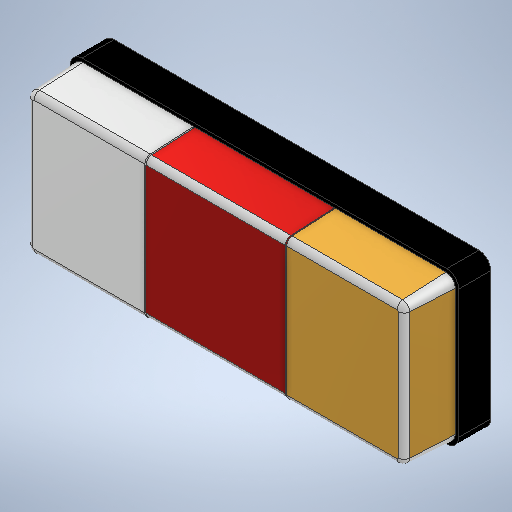
# Autodesk Inventor part: Arjun_RearLight
Saved by Autodesk Inventor 2025 (Build 290162000, 162)
## iProperties
Created: 2024-11-03
Part Number: Arjun_RearLight
Material: Generic
Document SubType Name: Modeling
Designer: pathl
Density: 1 g/cm^3
Appearance: Default
Author: pathl
Autodesk Inventor part; units mm, degrees
ref_plane "YZ Plane" through (0, 0, 0) normal (1, 0, 0) x (0, 1, 0)
ref_plane "XZ Plane" through (0, 0, 0) normal (0, 1, 0) x (-1, 0, 0)
ref_plane "XY Plane" through (0, 0, 0) normal (0, 0, 1) x (1, 0, 0)
sketch "Sketch1" plane through (0, 0, 0) normal (0, 0, 1) x (1, 0, 0)
  line L0 (7, 90) -> (223, 90)
  line L1 (230, 83) -> (230, 7)
  line L2 (223, 0) -> (7, 0)
  line L3 (0, 7) -> (0, 83)
  arc A0 (0, 7) -> (7, 0) centre (7, 7) ccw
  arc A1 (7, 90) -> (0, 83) centre (7, 83) ccw
  arc A2 (230, 83) -> (223, 90) centre (223, 83) ccw
  arc A3 (223, 0) -> (230, 7) centre (223, 7) ccw
  point P0 (0, 0)
  point P1 (0, 90)
  point P2 (230, 90)
  dimension "d0" = 230
  dimension "d1" = 90
  dimension "d2" = 7
  constraints: 8 end point, 8 point on circle, 8 tangent, 4 centre point, 4 point on line, 3 equal radius, 2 parallel, 1 horizontal, 1 perpendicular
  measures "d0" distance of point (0, 90) point (230, 90)
  measures "d1" distance between parallel lines of L2 L0
  measures "d2" radius of A0
extrude "Extrusion1" add sketch "Sketch1" along normal blind 19
sketch "Sketch2" plane through (0, 0, 19) normal (0, 0, 1) x (1, 0, 0)
  line L0 (7.5, 86.5) -> (222.5, 86.5)
  line L1 (226.5, 82.5) -> (226.5, 7.5)
  line L2 (230, 7) -> (230, 83) projected
  line L3 (222.5, 3.5) -> (7.5, 3.5)
  line L4 (3.5, 7.5) -> (3.5, 82.5)
  line L5 (223, 90) -> (7, 90) projected
  line L6 (7, 0) -> (223, 0) projected
  line L7 (0, 83) -> (0, 7) projected
  arc A0 (7.5, 86.5) -> (3.5, 82.5) centre (7.5, 82.5) ccw
  arc A1 (3.5, 7.5) -> (7.5, 3.5) centre (7.5, 7.5) ccw
  arc A2 (226.5, 82.5) -> (222.5, 86.5) centre (222.5, 82.5) ccw
  arc A3 (222.5, 3.5) -> (226.5, 7.5) centre (222.5, 7.5) ccw
  line L8 (73.1001, 86.5) -> (157.0688, 86.5)
  line L9 (157.0688, 86.5) -> (157.0688, 3.5)
  line L10 (157.0688, 3.5) -> (73.1001, 3.5)
  line L11 (73.1001, 3.5) -> (73.1001, 86.5)
  point P0 (0, 0)
  point P1 (73.1001, 3.5)
  dimension "d5" = 3.5
  dimension "d6" = 3.5
  dimension "d7" = 3.5
  dimension "d8" = 3.5
  dimension "d9" = 4
  dimension "d10" = 4
  constraints: 16 end point, 8 point on circle, 8 tangent, 4 centre point, 3 parallel, 3 perpendicular, 2 equal radius, 2 horizontal, 2 point on line
  measures "d5" distance between parallel lines of L0 L5
  measures "d6" distance between parallel lines of L2 L1
  measures "d7" distance between parallel lines of L6 L3
  measures "d8" distance between parallel lines of L7 L4
  measures "d9" radius of A0
  measures "d10" radius of A1
sketch "Sketch3" plane through (0, 0, 19) normal (0, 0, 1) x (1, 0, 0)
  line L0 (73.8321, 86.4013) -> (156.378, 86.4013)
  line L1 (156.378, 86.4013) -> (156.378, 3.8554)
  line L2 (156.378, 3.8554) -> (73.8321, 3.8554)
  line L3 (73.8321, 3.8554) -> (73.8321, 86.4013)
  point P0 (0, 0)
  constraints: 8 end point, 2 parallel, 1 horizontal, 1 perpendicular
sketch "Sketch4" plane through (0, 0, 19) normal (0, 0, 1) x (1, 0, 0)
  point P0 (0, 0)
extrude "Extrusion2" add sketch "Sketch3" along normal blind 29
extrude "Extrusion3" add sketch "Sketch2" along normal blind 29 contours L0 L11 L3 A1 L4 A0 | L0 A2 L1 A3 L3 L9
draft "FaceDraft1" angle 3 pull direction (0, 0, 1) faces at (101.3474, 3.8554, 28.6667) (178.8792, 3.5, 28.6667) (222.7989, 3.5112, 28.6667) (226.5, 32.5, 28.6667) (226.3223, 83.679, 38.3333) (200.6896, 86.5, 28.6667) (29.3667, 3.5, 28.6667) (4.0359, 5.5, 38.3333) (3.5, 57.5, 28.6667) (5.2467, 85.805, 38.3333) (51.2334, 86.5, 28.6667) (128.8627, 86.4013, 28.6667) fixed edges at (115.105, 3.8554, 48) (189.7844, 3.5, 48) (225.3284, 4.6716, 48) (226.5, 45, 48) (225.3284, 85.3284, 48) (189.7844, 86.5, 48) (40.3, 3.5, 48) (4.6716, 4.6716, 48) (3.5, 45, 48) (4.6716, 85.3284, 48) (40.3, 86.5, 48) (115.105, 86.4013, 48)
fillet "Fillet1" radius 3.5 12 edges at (115.105, 3.8554, 48) (225.3284, 4.6716, 48) (226.5, 45, 48) (225.3284, 85.3284, 48) (189.7844, 86.5, 48) (189.7844, 3.5, 48) (115.105, 86.4013, 48) (4.6716, 85.3284, 48) (3.5, 45, 48) (4.6716, 4.6716, 48) (40.3, 3.5, 48) (40.3, 86.5, 48)
body "Solid1"
